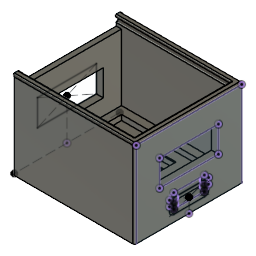
3d enclosure (Autodesk Fusion 360 design; units mm, degrees)
part number: 2026-02-15-22-55-38-721
part number: 2026-02-16-00-24-04-871
Autodesk Fusion 360 part; units mm, degrees
note: some values were not read from the file. Chosen so that the rebuilt part matches the saved one: that a step has no effect; which pieces of a blend or face edit are solid.
sketch "base" plane through (0, 0, 0) normal (0, 0, 1) x (1, 0, 0) in component "main cover"
  line L0 (14, -12.5) -> (-14, -12.5)
  line L1 (-14, -12.5) -> (-14, 12.5)
  line L2 (-14, 12.5) -> (14, 12.5)
  line L3 (14, 12.5) -> (14, -12.5)
  line L4 (14, -12.5) -> (-14, 12.5) construction
  line L5 (-14, -12.5) -> (14, 12.5) construction
  dimension "d15" = 28
  dimension "d16" = 25
  constraint horizontal L0
  constraint perpendicular L0 L1
  constraint parallel L0 L2
  constraint parallel L1 L3
  constraint coincident L4 origin
  constraint coincident L5 origin
  measures "d15" distance of L1.end L2.end
  measures "d16" distance of L0.end L1.end
extrude "Extrude1" add sketch "base" along normal blind 20 makes body 1 in component "main cover"
shell "Shell1" thickness 1.6 removed faces 1 at (4.6667, -4.1667, 20) on bodies 1 in component "main cover"
sketch "usb port" plane through (14, 0, 0) normal (1, 0, 0) x (0, 1, 0) in component "main cover"
  line L0 (-12.5, 0) -> (12.5, 0)
  line L1 (12.5, 0) -> (12.5, 20)
  line L2 (12.5, 20) -> (-12.5, 20)
  line L3 (-12.5, 20) -> (-12.5, 0)
  line L4 (0, 0) -> (0, 2.6)
  line L5 (0, 2.6) -> (0, 4.25)
  line L6 (-3.5, 2.6) -> (3.5, 2.6)
  line L7 (4.5, 3.6) -> (4.5, 4.9)
  line L8 (3.5, 5.9) -> (-3.5, 5.9)
  line L9 (-4.5, 4.9) -> (-4.5, 3.6)
  line L10 (-4.5, 2.6) -> (4.5, 5.9) construction
  line L11 (4.5, 2.6) -> (-4.5, 5.9) construction
  arc A0 (4.5, 4.9) -> (3.5, 5.9) centre (3.5, 4.9) ccw
  arc A1 (-4.5, 3.6) -> (-3.5, 2.6) centre (-3.5, 3.6) ccw
  arc A2 (-3.5, 5.9) -> (-4.5, 4.9) centre (-3.5, 4.9) ccw
  arc A3 (3.5, 2.6) -> (4.5, 3.6) centre (3.5, 3.6) ccw
  point P0 (0, 4.25)
  dimension "d26" = 2.6
  dimension "d27" = 1.65
  dimension "d28" = 9
  dimension "d29" = 3.3
  dimension "d30" = 1
  constraint coincident L4.start origin
  constraint perpendicular L0 L4
  constraint parallel L4 L5
  constraint horizontal L6
  constraint perpendicular L6 L7
  constraint parallel L6 L8
  constraint parallel L7 L9
  constraint coincident L10 P0
  constraint coincident L11 P0
  constraint coincident P0 L5.end
  constraint coincident L10.end L8
  constraint coincident L10.end L7
  constraint tangent L8 A0
  constraint tangent L7 A0
  constraint coincident L10.start L6
  constraint coincident L10.start L9
  constraint tangent L6 A1
  constraint tangent L9 A1
  constraint equal A0 A1
  constraint coincident L11.end L9
  constraint coincident L11.end L8
  constraint tangent L9 A2
  constraint tangent L8 A2
  constraint equal A0 A2
  constraint coincident L11.start L7
  constraint coincident L11.start L6
  constraint tangent L7 A3
  constraint tangent L6 A3
  constraint equal A0 A3
  measures "d26" distance of L4.start L4.end
  measures "d27" distance of L4.end P0
  measures "d28" distance of L10.end L11.end
  measures "d29" distance of L11.start L10.end
  measures "d30" radius of A0
extrude "Extrude2" cut sketch "usb port" against normal blind 1.698 contours L6 L7 L8 L9 A0 A1 A2 A3 bodies 1 in component "main cover"
sketch "esp support" plane through (0, 0, 1.6) normal (0, 0, 1) x (-1, 0, 0) in component "main cover"
  line L0 (-12.4, -10.9) -> (12.4, -10.9)
  line L1 (12.4, -10.9) -> (12.4, 10.9)
  line L2 (12.4, 10.9) -> (-12.4, 10.9)
  line L3 (-12.4, 10.9) -> (-12.4, -10.9)
  line L4 (-12.4, -10.9) -> (-12.4, 10.9)
  line L5 (-12.4, 10.9) -> (12.4, 10.9)
  line L6 (12.4, 10.9) -> (12.4, -10.9)
  line L7 (12.4, -10.9) -> (-12.4, -10.9)
  line L8 (-14, 12.5) -> (-14, -12.5)
  line L9 (-14, -12.5) -> (14, -12.5)
  line L10 (14, -12.5) -> (14, 12.5)
  line L11 (14, 12.5) -> (-14, 12.5)
  line L12 (-11.4, -9.9) -> (-11.4, 9.9)
  line L13 (-11.4, 9.9) -> (11.4, 9.9)
  line L14 (11.4, 9.9) -> (11.4, -9.9)
  line L15 (11.4, -9.9) -> (-11.4, -9.9)
  dimension "d33" = 1
extrude "Extrude3" add sketch "esp support" along normal blind 0.4 separate body contours L0 L1 L2 L3 L4 L5 L6 L7 makes body 2 in component "main cover"
extrude "Extrude4" add 1 faces at (-11.4, -3.3, 1.7333) along direction (1, 0, 0) blind 3 on bodies 2 bodies 2 in component "main cover"
extrude "Extrude5" cut 1 faces at (-8.4, -3.3, 1.7333) along direction (-1, 0, 0) blind 3.72 on bodies 2 bodies 2 in component "main cover"
extrude "Extrude6" cut 1 faces at (11.4, 3.3, 1.7333) along direction (1, 0, 0) blind 1 on bodies 2 bodies 2 in component "main cover"
extrude "Extrude7" add 1 faces at (-12.12, -3.3, 1.7333) along direction (1, 0, 0) blind 1 on bodies 2 bodies 2 in component "main cover"
extrude "Extrude8" add 1 faces at (-11.12, -3.3, 1.7333) along direction (1, 0, 0) blind 0.5 on bodies 2 bodies 1 2 in component "main cover"
extrude "Extrude9" add 1 faces at (-2.9467, 9.9, 1.7333) along direction (0, -1, 0) blind 0.75 on bodies 1 bodies 1 in component "main cover"
extrude "Extrude10" add 1 faces at (-2.9467, -9.9, 1.7333) along direction (0, 1, 0) blind 0.75 on bodies 1 bodies 1 in component "main cover"
sketch "output usb " plane through (14, 0, 0) normal (1, 0, 0) x (0, 1, 0) in component "main cover"
  line L0 (4.5, 4.9) -> (4.5, 3.6)
  arc A0 (3.5, 2.6) -> (4.5, 3.6) centre (3.5, 3.6) ccw
  line L1 (3.5, 2.6) -> (-3.5, 2.6)
  arc A1 (-4.5, 3.6) -> (-3.5, 2.6) centre (-3.5, 3.6) ccw
  line L2 (-4.5, 3.6) -> (-4.5, 4.9)
  arc A2 (-3.5, 5.9) -> (-4.5, 4.9) centre (-3.5, 4.9) ccw
  line L3 (-3.5, 5.9) -> (3.5, 5.9)
  arc A3 (4.5, 4.9) -> (3.5, 5.9) centre (3.5, 4.9) ccw
  line L4 (-12.5, 0) -> (12.5, 0)
  line L5 (12.5, 0) -> (12.5, 20)
  line L6 (12.5, 20) -> (-12.5, 20)
  line L7 (-12.5, 20) -> (-12.5, 0)
  line L8 (3.5, 5.9) -> (-3.5, 5.9)
  line L9 (-3.5, 5.9) -> (3.5, 5.9)
  line L10 (0, 5.9) -> (0, 11.4) construction
  line L11 (6.75, 14.4) -> (-6.75, 14.4)
  line L12 (-6.75, 14.4) -> (-6.75, 8.4)
  line L13 (-6.75, 8.4) -> (6.75, 8.4)
  line L14 (6.75, 8.4) -> (6.75, 14.4)
  line L15 (6.75, 14.4) -> (-6.75, 8.4) construction
  line L16 (-6.75, 14.4) -> (6.75, 8.4) construction
  point P0 (0, 4.25)
  point P1 (4.5, 4.9)
  point P2 (3.5, 5.9)
  point P3 (-3.5, 5.9)
  point P4 (0, 11.4)
  dimension "d50" = 5.5
  dimension "d51" = 13.5
  dimension "d52" = 6
  constraint coincident P3 A2.start
  constraint coincident P2 L3.end
  constraint midpoint L8 L10.start
  constraint perpendicular L8 L10
  constraint horizontal L11
  constraint perpendicular L11 L12
  constraint parallel L11 L13
  constraint parallel L12 L14
  constraint coincident L15 P4
  constraint coincident L16 P4
  constraint coincident P4 L10.end
  measures "d50" distance of L10.start P4
  measures "d51" distance of L12.end L13.end
  measures "d52" distance of L11.end L12.end
extrude "Extrude11" cut sketch "output usb " against normal blind 1.6 contours L11 L12 L13 L14 bodies 1 in component "main cover"
sketch "lid opening" plane through (-12.4, 0, 0) normal (1, 0, 0) x (0, 1, 0) in component "main cover"
  line L0 (-10.9, 2) -> (10.9, 2)
  line L1 (10.9, 2) -> (10.9, 20)
  line L2 (10.9, 20) -> (-10.9, 20)
  line L3 (-10.9, 20) -> (-10.9, 2)
  line L4 (12.5, 20) -> (-12.5, 20)
  line L5 (12.5, 0) -> (-12.5, 0)
  line L6 (-12.5, 0) -> (-12.5, 20)
  line L7 (-12.5, 20) -> (12.5, 20)
  line L8 (12.5, 20) -> (12.5, 0)
  line L9 (10.9, 20) -> (10.9, 18)
  line L10 (10.9, 18) -> (-10.9, 18)
  dimension "d55" = 2
  constraint coincident L1.end L2.start
  constraint perpendicular L4 L9
  constraint coincident L3 L10.end
  constraint perpendicular L3 L10
  measures "d55" distance of L1.end L9.end
extrude "Extrude12" cut sketch "lid opening" against normal blind 1.6 contours L1 L2 L3 L4 L7 L9 L10 bodies 1 in component "main cover"
sketch "Sketch8" plane through (0, -10.9, 0) normal (0, 1, 0) x (-1, 0, 0) in component "main cover"
  line L0 (-12.4, 2) -> (12.4, 2)
  line L1 (12.4, 2) -> (12.4, 18)
  line L2 (12.4, 18) -> (14, 18)
  line L3 (14, 18) -> (14, 20)
  line L4 (14, 20) -> (-12.4, 20)
  line L5 (-12.4, 20) -> (-12.4, 2)
  line L6 (14, 20) -> (14, 18.4)
  line L7 (14, 19.2) -> (-12.4, 19.2)
  line L8 (-12.4, 19.2, 0) -> (-12.4, 19.2, 21.8)
  line L9 (-12.4, 2, 21.8) -> (-12.4, 20, 21.8)
  line L10 (14, 18, 21.8) -> (14, 20, 21.8)
  line L11 (-12.4, 19.2, 21.8) -> (14, 19.2, 21.8)
  line L12 (14, 20, 21.8) -> (-12.4, 20, 21.8)
  line L13 (-12.4, 20, 21.8) -> (-12.4, 20, 0)
  line L14 (-0.0144, 19.2, 21.8) -> (-0.0144, 20, 21.8)
  line L15 (14, 19.2, 21.8) -> (14, 19.7, 21.8) construction
  line L16 (14, 19.2, 21.8) -> (14, 18.7, 21.8) construction
  dimension "d58" = 1.6
  dimension "d59" = 0.5
  dimension "d60" = 0.5
  constraint coincident L3.end L4.start
  constraint coincident L3 L6.end
  constraint midpoint L6 L7.start
  constraint coincident L5 L7.end
  constraint perpendicular L5 L7
  constraint coincident L7.end
  measures "d58" distance of L3.end L6.end
sketch "Sketch10" plane through (-14, 0, 0) normal (-1, 0, 0) x (0, -1, 0) in component "main cover"
  line L0 (-10.9, 18) -> (-10.9, 20)
  line L1 (-10.9, 20) -> (-12.5, 20)
  line L2 (-12.5, 20) -> (-12.5, 0)
  line L3 (-12.5, 0) -> (12.5, 0)
  line L4 (12.5, 0) -> (12.5, 20)
  line L5 (12.5, 20) -> (10.9, 20)
  line L6 (10.9, 20) -> (10.9, 18)
  line L7 (10.9, 18) -> (-10.9, 18)
  arc A0 (-10.9, 19.7127) -> (-10.9, 18.7127) centre (-10.9, 19.2127) ccw
  dimension "d67" = 0.5
  constraint coincident L0 A0.start
  constraint coincident L0 A0.centre
  measures "d67" radius of A0
sweep "Sweep2" cut profiles "Sketch10" path "Sketch8" along L7 L8 L11 section 1 contours L0 A0 bodies 1 in component "main cover"
sketch "Sketch1" plane through (-14, 0, 0) normal (-1, 0, 0) x (0, -1, 0)
  line L0 (-10.9, 19.7) -> (-10.9, 20)
  line L1 (10.9, 20.0001) -> (10.9, 20)
  line L2 (-10.9, 20) -> (10.9, 20) construction
  line L3 (-10.9, 18) -> (10.9, 18) construction
  line L4 (0, 20) -> (0, 18) construction
  point P0 (-10.9, 19.2)
  point P1 (-10.9, 19.7)
  point P2 (-10.9, 18.7127)
  point P3 (10.9, 20)
  point P4 (10.9, 18)
  constraint coincident P1 L0.start
  constraint coincident P3 L1.end
  constraint coincident P4 L3.end
  constraint midpoint L2 L4.start
  constraint midpoint L3 L4.end
fillet "Fillet1" radius 0.4 2 edges at (-14, -12.5, 10) (0, -12.5, 20) on bodies 1 in component "main cover"
fillet "Fillet1" radius 0.4 13 edges at (14, -12.5, 10) (14, 12.5, 10) (-14, 12.5, 10) (0, 12.5, 20) (14, 0, 20) (-0.8, -10.9, 20) (-0.8, 10.9, 20) (12.4, 0, 20) (-14, -10.9, 18.3564) (-14, -11.4, 19.2127) (-14, 0, 18) (-14, 10.9, 18.3564) (-14, 11.4, 19.2127) on bodies 1 in component "main cover"
extrude "Extrude13" add 1 faces at (-11.8067, -3.05, 2) along direction (0, 0, 1) blind 0.8 on bodies 1 bodies 1 in component "main cover"
sketch "Sketch2" plane through (0, 0, 2.8) normal (0, 0, 1) x (-1, 0, 0)
  line L0 (-12.4, -9.15) -> (-12.4, -10.9)
  line L1 (-12.4, -10.9) -> (12.4, -10.9)
  line L2 (12.4, -10.9) -> (12.4, 10.9)
  line L3 (12.4, 10.9) -> (-12.4, 10.9)
  line L4 (-12.4, 10.9) -> (-12.4, 9.15)
  line L5 (-12.4, 9.15) -> (10.62, 9.15)
  line L6 (10.62, 9.15) -> (10.62, -9.15)
  line L7 (10.62, -9.15) -> (-12.4, -9.15)
sketch "Sketch3" plane through (0, 0, 1.6) normal (0, 0, 1) x (-1, 0, 0)
  line L0 (10.62, 9.15) -> (-12.4, 9.15)
  line L1 (-12.4, 9.15) -> (-12.4, -9.15)
  line L2 (-12.4, -9.15) -> (10.62, -9.15)
  line L3 (10.62, -9.15) -> (10.62, 9.15)
  line L4 (10.62, 9.15) -> (10.62, -9.15) construction
  line L5 (-3.88, -0.0025) -> (-3.88, -7.0011) construction
  line L6 (10.62, -6.9961) -> (10.62, 7.5039)
  line L7 (10.62, -6.9961) -> (-3.88, -6.9961)
  line L8 (-3.88, -6.9961) -> (-3.88, 7.4989)
  line L9 (-3.88, 7.4989) -> (10.62, 7.4989)
  line L10 (10.62, 7.4989) -> (10.62, -6.9961)
  line L11 (10.62, -6.9961) -> (-3.88, -6.9961)
  line L12 (-3.88, -6.9961) -> (-3.88, -6.3461)
  line L13 (-3.88, -6.3461) -> (10.62, -6.3461)
  line L14 (10.62, -6.3461) -> (10.62, -6.9961)
  line L15 (-3.88, -4.0377) -> (10.62, -4.0377)
  line L16 (10.62, -4.6877) -> (-3.88, -4.6877)
  line L17 (-3.88, -1.7294) -> (10.62, -1.7294)
  line L18 (10.62, -2.3794) -> (-3.88, -2.3794)
  line L19 (-3.88, 0.5789) -> (10.62, 0.5789)
  line L20 (10.62, -0.0711) -> (-3.88, -0.0711)
  line L21 (-3.88, 2.8873) -> (10.62, 2.8873)
  line L22 (10.62, 2.2373) -> (-3.88, 2.2373)
  line L23 (-3.88, 5.1956) -> (10.62, 5.1956)
  line L24 (10.62, 4.5456) -> (-3.88, 4.5456)
  line L25 (-3.88, 7.5039) -> (10.62, 7.5039)
  line L26 (10.62, 6.8539) -> (-3.88, 6.8539)
  dimension "d84" = 14.5
  dimension "d88" = 14.5
  dimension "d90" = 0.65
  dimension "d93" = -0.5
  dimension "d94" = 13.85
  constraint coincident L0.start L3.end
  constraint coincident L2.end L3.start
  constraint coincident L3 L6.start
  constraint coincident L3 L6.end
  constraint horizontal L7
  constraint vertical L8
  constraint horizontal L9
  constraint vertical L10
  constraint vertical L5
  constraint horizontal L11
  constraint vertical L12
  constraint horizontal L13
  constraint vertical L14
  constraint coincident L5 L12.end
  measures "d84" distance of L6.start L6.end
  measures "d88" distance of L6.start L7.end
  measures "d90" distance of L6.start L13.end
extrude "Extrude14" cut sketch "Sketch3" against normal blind 2 contours L3 L6 L8 L9 L10 L26 | L3 L6 L7 L8 L10 L11 L12 L13 L14 | L3 L6 L8 L10 L23 L24 | L3 L6 L8 L10 L15 L16 | L3 L6 L8 L10 L21 L22 | L3 L6 L8 L10 L17 L18 | L3 L6 L8 L10 L19 L20 bodies 1 in component "main cover"
extrude "Extrude15" cut sketch "Sketch3" against normal blind 0.5 contours L3 L6 L8 L10 L23 L26 | L3 L6 L8 L10 L13 L16 | L3 L6 L8 L10 L21 L24 | L3 L6 L8 L10 L15 L18 | L3 L6 L8 L10 L19 L22 | L3 L6 L8 L10 L17 L20 bodies 1 in component "main cover"
fillet "Fillet2" radius 0.15 14 edges at (-3.37, 6.3461, 1.1) (-3.37, 4.6877, 1.1) (-3.37, 4.0377, 1.1) (-3.37, 2.3794, 1.1) (-3.37, 1.7294, 1.1) (-3.37, 0.0711, 1.1) (-3.37, -0.5789, 1.1) (-3.37, -2.2373, 1.1) (-3.37, -2.8873, 1.1) (-3.37, -4.5456, 1.1) (-3.37, -5.1956, 1.1) (-3.37, -6.8539, 1.1) (-3.37, -7.4989, 1.6) (-3.37, 6.9961, 1.6) on bodies 1 in component "main cover"
sketch "Sketch5" plane through (-14, 0, 0) normal (-1, 0, 0) x (0, -1, 0)
  arc A0 (-11.3361, 20) -> (-11.3, 18.4065) centre (-10.9, 19.2127) ccw
  line L0 (-11.3361, 20) -> (-12.1, 20)
  line L1 (-12.1, 20) -> (-12.1, 0)
  line L2 (-12.1, 0) -> (12.1, 0)
  line L3 (12.1, 0) -> (12.1, 20)
  line L4 (12.1, 20) -> (11.3361, 20)
  arc A1 (11.3, 18.4065) -> (11.3361, 20) centre (10.9, 19.2127) ccw
  line L5 (11.3, 18.4065) -> (11.3, 17.6)
  line L6 (11.3, 17.6) -> (-11.3, 17.6)
  line L7 (-11.3, 17.6) -> (-11.3, 18.4065)
  line L8 (-12.1, 0) -> (12.1, 0) construction
  line L9 (0, 0) -> (0, 9.4) construction
  line L10 (6.75, 12.4) -> (-6.75, 12.4)
  line L11 (-6.75, 12.4) -> (-6.75, 6.4)
  line L12 (-6.75, 6.4) -> (6.75, 6.4)
  line L13 (6.75, 6.4) -> (6.75, 12.4)
  line L14 (6.75, 12.4) -> (-6.75, 6.4) construction
  line L15 (-6.75, 12.4) -> (6.75, 6.4) construction
  point P0 (0, 9.4)
  dimension "d101" = 9.4
  dimension "d102" = 13.5
  dimension "d103" = 6
  constraint coincident L1.end L2.start
  constraint coincident L2.end L3.start
  constraint coincident L9.start origin
  constraint perpendicular L8 L9
  constraint horizontal L10
  constraint perpendicular L10 L11
  constraint parallel L10 L12
  constraint parallel L11 L13
  constraint coincident L14 P0
  constraint coincident L15 P0
  constraint coincident P0 L9.end
  measures "d101" distance of L9.start P0
  measures "d102" distance of L11.end L12.end
  measures "d103" distance of L10.end L11.end
extrude "Extrude16" cut sketch "Sketch5" against normal blind 2 contours L10 L11 L12 L13 bodies 1 in component "main cover"
sweep "Sweep1" [no effect] in component "main cover"
sketch "Sketch2 (2)" plane through (14, 0, 0) normal (1, 0, 0) x (0, 1, 0) in component "main cover"
  line L0 (-12.1, 0) -> (12.1, 0)
  line L1 (0, 0) -> (0, 1.6) construction
  line L2 (0, 1.6) -> (0, 3.25) construction
  line L3 (-3.5, 4.9) -> (3.5, 4.9)
  line L4 (4.5, 3.9) -> (4.5, 2.6)
  line L5 (3.5, 1.6) -> (-3.5, 1.6)
  line L6 (-4.5, 2.6) -> (-4.5, 3.9)
  line L7 (-4.5, 4.9) -> (4.5, 1.6) construction
  line L8 (4.5, 4.9) -> (-4.5, 1.6) construction
  arc A0 (-3.5, 4.9) -> (-4.5, 3.9) centre (-3.5, 3.9) ccw
  arc A1 (4.5, 3.9) -> (3.5, 4.9) centre (3.5, 3.9) ccw
  arc A2 (3.5, 1.6) -> (4.5, 2.6) centre (3.5, 2.6) ccw
  arc A3 (-4.5, 2.6) -> (-3.5, 1.6) centre (-3.5, 2.6) ccw
  line L9 (12.1, 0) -> (12.1, 19.6)
  line L10 (12.1, 19.6) -> (-12.1, 19.6)
  line L11 (-12.1, 19.6) -> (-12.1, 0)
  line L12 (4.5, 4.9) -> (4.5, 3.6)
  arc A4 (3.5, 2.6) -> (4.5, 3.6) centre (3.5, 3.6) ccw
  line L13 (3.5, 2.6) -> (-3.5, 2.6)
  arc A5 (-4.5, 3.6) -> (-3.5, 2.6) centre (-3.5, 3.6) ccw
  line L14 (-4.5, 3.6) -> (-4.5, 4.9)
  arc A6 (-3.5, 5.9) -> (-4.5, 4.9) centre (-3.5, 4.9) ccw
  line L15 (-3.5, 5.9) -> (3.5, 5.9)
  arc A7 (4.5, 4.9) -> (3.5, 5.9) centre (3.5, 4.9) ccw
  line L16 (-6.75, 14.4) -> (6.75, 14.4)
  line L17 (6.75, 14.4) -> (6.75, 8.4)
  line L18 (6.75, 8.4) -> (-6.75, 8.4)
  line L19 (-6.75, 8.4) -> (-6.75, 14.4)
  point P0 (0, 3.25)
  dimension "d20" = 1.6
  dimension "d22" = 1.65
  dimension "d23" = 9
  dimension "d24" = 3.3
  dimension "d25" = 1
  constraint coincident L1.start origin
  constraint perpendicular L0 L1
  constraint parallel L1 L2
  constraint horizontal L3
  constraint perpendicular L3 L4
  constraint parallel L3 L5
  constraint parallel L4 L6
  constraint coincident L7 P0
  constraint coincident L8 P0
  constraint coincident P0 L2.end
  constraint coincident L7.start L6
  constraint coincident L7.start L3
  constraint tangent L6 A0
  constraint tangent L3 A0
  constraint coincident L8.start L3
  constraint coincident L8.start L4
  constraint tangent L3 A1
  constraint tangent L4 A1
  constraint equal A0 A1
  constraint coincident L7.end L4
  constraint coincident L7.end L5
  constraint tangent L4 A2
  constraint tangent L5 A2
  constraint equal A0 A2
  constraint coincident L8.end L5
  constraint coincident L8.end L6
  constraint tangent L5 A3
  constraint tangent L6 A3
  constraint equal A0 A3
  measures "d20" distance of L1.start L1.end
  measures "d22" distance of L1.end P0
  measures "d23" distance of L7.end L8.end
  measures "d24" distance of L8.start L7.end
  measures "d25" radius of A0
component "main cover" placed x (1, 0, 0) y (0, 1, 0) z (0, 0, 1) at (0, 0, 0)
named bodies: "esp placeholder"
